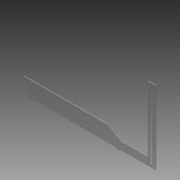
# Autodesk Inventor part: Side Wall 2
Saved by Autodesk Inventor 2013 (Build 170138000, 138)
## iProperties
Created: 2013-01-28
Part Number: Side Wall 2
Material: Polycarbonate, Clear
Document SubType Name: Modeling
Designer: Andrew Toennies
Density: 1.2 g/cm^3
Mass: 92.2992 g
Surface Area: 542.895 cm^2
Volume: 76.916 cm^3
Author: Andrew Toennies
Autodesk Inventor part; units mm, degrees
ref_plane "YZ Plane" through (0, 0, 0) normal (1, 0, 0) x (0, 1, 0)
ref_plane "XZ Plane" through (0, 0, 0) normal (0, 1, 0) x (-1, 0, 0)
ref_plane "XY Plane" through (0, 0, 0) normal (0, 0, 1) x (1, 0, 0)
sketch "Sketch1" plane through (0, 0, 0) normal (0, 0, 1) x (1, 0, 0)
  line L0 (0, 0) -> (3.175, 0)
  line L1 (3.175, 0) -> (3.175, -3.175)
  line L2 (3.175, -3.175) -> (15.875, -3.175)
  line L3 (15.875, -3.175) -> (15.875, 0)
  line L4 (0, 0) -> (0, 25.4)
  line L5 (307.975, 0) -> (15.875, 0)
  line L6 (0, 25.4) -> (-11.8442, 50.8)
  line L7 (307.975, 25.4) -> (263.9809, 50.8)
  line L8 (-11.8442, 50.8) -> (263.9809, 50.8)
  line L9 (358.775, 0) -> (422.275, 0)
  line L10 (307.975, 0) -> (358.775, 0)
  line L11 (307.975, 25.4) -> (384.175, 25.4)
  line L12 (384.175, 25.4) -> (384.175, 241.3)
  line L13 (384.175, 241.3) -> (422.275, 241.3)
  line L14 (422.275, 241.3) -> (422.275, 0)
  line L15 (588.0391, 190.1261) -> (586.2287, 190.1261) projected
  line L16 (586.2287, 218.7011) -> (586.2287, 190.1261) projected
  line L17 (588.0391, 218.7011) -> (586.2287, 218.7011) projected
  line L18 (588.0391, 190.1261) -> (588.0391, 218.7011) projected
  line L19 (588.0391, 38.1) -> (586.2287, 38.1) projected
  line L20 (586.2287, 177.4261) -> (586.2287, 38.1) projected
  line L21 (586.2287, 177.4261) -> (588.0391, 177.4261) projected
  line L22 (588.0391, 38.1) -> (588.0391, 177.4261) projected
  line L23 (588.0391, 190.1261) -> (588.0391, 218.7011) projected
  line L24 (588.0391, 190.1261) -> (586.2287, 190.1261) projected
  line L25 (586.2287, 218.7011) -> (586.2287, 190.1261) projected
  line L26 (588.0391, 218.7011) -> (586.2287, 218.7011) projected
  line L27 (588.0391, 190.1261) -> (588.0391, 218.7011) projected
  line L28 (431.5435, 218.7011) -> (431.5435, 12.7) projected
  line L29 (431.5435, 218.7011) -> (429.7331, 218.7011) projected
  line L30 (429.7331, 12.7) -> (429.7331, 218.7011) projected
  line L31 (431.5435, 12.7) -> (429.7331, 12.7) projected
  dimension "d0" = 3.175
  dimension "d1" = 3.175
  dimension "d2" = 12.7
  dimension "d3" = 25.4
  dimension "d4" = 307.975
  dimension "d12" = 25.4
  dimension "d13" = 25
  dimension "d17" = 25.4
  dimension "d19" = 150
  dimension "d21" = 25.4
  dimension "d25" = 0
  dimension "d36" = 215.9
  dimension "d37" = 38.1
  dimension "d44" = 76.2
  constraints: 30 end point, 7 parallel, 2 horizontal, 2 perpendicular, 1 collinear
  measures "d0" distance of L0.start L0.end
  measures "d1" distance of L0.end L1.end
  measures "d2" distance of L1.end L2.end
  measures "d3" distance of L0.start L4.end
  measures "d4" distance of L4.end L7.start
  measures "d12" distance from line of L8 L4.end
  measures "d13" angle of L6 L4
  measures "d17" distance of L5.start L7.start
  measures "d19" angle of L8 L7
  measures "d21" vertical distance of L7.end L7.start
  measures "d25" vertical distance of L9.start L9.end
  measures "d36" distance of L11.end L12.end
  measures "d37" distance of L12.end L13.end
  measures "d44" distance of L7.start L11.end
extrude "Extrusion1" add sketch "Sketch1" along normal blind 3.175 contours L4 L6 L8 L7 L11 L12 L13 L14 L9 L10 L5 L3 L2 L1 L0
sketch "Sketch2" plane through (0, 0, 3.175) normal (0, 0, 1) x (1, 0, 0)
  line L0 (289.5902, 0) -> (302.2902, 0) projected
  line L1 (289.5902, -3.175) -> (289.5902, 0) projected
  line L2 (302.2902, -3.175) -> (289.5902, -3.175) projected
  line L3 (302.2902, 0) -> (302.2902, -3.175) projected
extrude "Extrusion2" add sketch "Sketch2" against normal blind 3.175
sketch "Sketch3" plane through (0, 0, 0) normal (0, 0, -1) x (-1, 0, 0)
  line L0 (-384.175, 241.3) -> (-384.175, 25.4) projected
  line L1 (-302.2902, 0) -> (-422.275, 0) projected
  line L2 (-397.7005, 225.425) -> (-397.7005, 9.525)
  line L3 (-397.7005, 9.525) -> (-407.9875, 9.525)
  line L4 (-407.9875, 9.525) -> (-407.9875, 225.425)
  line L5 (-407.9875, 225.425) -> (-397.7005, 225.425)
  line L6 (-422.275, 0) -> (-422.275, 241.3) projected
  dimension "d38" = 215.9
  dimension "d39" = 10.287
  dimension "d41" = 9.525
  dimension "d45" = 14.2875
  constraints: 8 end point, 2 parallel, 2 perpendicular
  measures "d38" distance of L2.start L2.end
  measures "d39" distance of L2.end L3.end
  measures "d41" distance between parallel lines of L1 L3
  measures "d45" distance between parallel lines of L6 L4
extrude "Extrusion3" cut sketch "Sketch3" against normal blind 25.4
body "Solid1"
